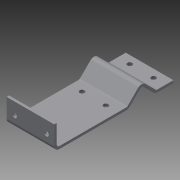
# Autodesk Inventor part: laserholder
Saved by Autodesk Inventor 2014 SP2 (Build 180246200, 246)
## iProperties
Created: 2016-05-15
Part Number: laserholder
Material: Generic
Document SubType Name: Sheet Metal
Designer: cruiser
Density: 1 g/cm^3
Sheet Metal Rule: Default_mm
Appearance: Default
Flat Pattern Width: 9.30164 cm
Flat Pattern Length: 3 cm
Flat Pattern Area: 27.9049 cm^2
Sheet Metal Width: 93.016 mm
Sheet Metal Length: 30.000 mm
Sheet Metal Area: 2790.493 mm^2
Author: cruiser
Autodesk Inventor part; units mm, degrees
ref_plane "YZ Plane" through (0, 0, 0) normal (1, 0, 0) x (0, 1, 0)
ref_plane "XZ Plane" through (0, 0, 0) normal (0, 1, 0) x (-1, 0, 0)
ref_plane "XY Plane" through (0, 0, 0) normal (0, 0, 1) x (1, 0, 0)
sketch "Sketch1" plane through (0, 0, 0) normal (0, 1, 0) x (-1, 0, 0)
  line L0 (15, -7.5) -> (-15, -7.5)
  line L1 (-15, -7.5) -> (-15, 7.5)
  line L2 (-15, 7.5) -> (15, 7.5)
  line L3 (15, 7.5) -> (15, -7.5)
  line L4 (15, -7.5) -> (-15, 7.5) construction
  line L5 (-15, -7.5) -> (15, 7.5) construction
  point P0 (0, 0)
  dimension "d10" = 30
  dimension "d11" = 15
  measures "d10" distance of L1.end L2.end
  measures "d11" distance of L0.end L1.end
extrude "Plate1" add sketch "Sketch1" along normal blind 1.5875
sketch "Sketch3" plane through (15, 0, 7.5) normal (1, 0, 0) x (0, 0, -1)
  line L0 (15, 0) -> (15, 1.5875)
  line L1 (15, 0) -> (15, 46.5147)
  line L2 (15, 0) -> (0, 0)
  line L3 (15, 63.4853) -> (15, 75)
  line L4 (6.5147, 55) -> (15, 46.5147)
  line L5 (15, 63.4853) -> (6.5147, 55)
  point P0 (7.5, 0)
  point P1 (15, 55)
  dimension "d48" = 75
  dimension "d91" = 55
  dimension "d92" = 0
  dimension "d94" = 90
  dimension "d95" = 135
  dimension "d96" = 6
  dimension "d97" = 6
  measures "d48" distance of L0.start L3.end
  measures "d91" distance from line of L2 point (15, 55)
  measures "d92" distance from line of L1 point (15, 55)
  measures "d94" angle of L5 L4
  measures "d95" angle of L3 L5
  measures "d96" distance from line of L4 point (15, 55)
  measures "d97" distance from line of L5 point (15, 55)
contour flange "Contour Flange4" sketch "Sketch3" thickness 1.5875 bend radius 1.5875 curves L1 L4 L5 L3 edges at (0, 1.5875, -7.5) running between points at (15, 1.5875, -7.5) (-15, 1.5875, -7.5)
bend "Bend4"
corner "Corner4"
sketch "Sketch4" plane through (-15, 75, -5.9125) normal (0, 0, 1) x (1, 0, 0)
  line L0 (0, -10.1996) -> (30, -10.1996) projected
  line L1 (30, 0) -> (0, 0) projected
  line L2 (0, 0) -> (0, -10.1996) projected
  circle A0 centre (7.5, -5) radius 1.5
  line L3 (15, 0) -> (15, -10.1996)
  circle A1 centre (22.5, -5) radius 1.5
  point P0 (15, -75)
  dimension "d50" = 3
  dimension "d52" = 5
  dimension "d53" = 7.5
  constraints: 2 centre point, 2 end point, 2 midpoint, 1 symmetric about line, 1 other
  measures "d50" diameter of A0
  measures "d52" distance from line of L1 A0.centre
  measures "d53" distance from line of L2 A0.centre
extrude "Cut1" cut sketch "Sketch4" against normal blind 1.5875 contours A0 | A1
sketch "Sketch9" plane through (-15, 45.1996, -5.9125) normal (0, 0, 1) x (1, 0, 0)
  line L0 (0, 0) -> (30, 0) projected
  line L1 (0, 0) -> (0, -42.0246) projected
  line L2 (0, -42.0246) -> (30, -42.0246) projected
  line L3 (30, 0) -> (30, -42.0246) projected
  circle A0 centre (7.5, -5.1996) radius 1.5
  line L4 (15, -42.0246) -> (15, 0)
  line L5 (0, -5.1996) -> (30, -5.1996)
  circle A1 centre (22.5, -5.1996) radius 1.5
  circle A2 centre (22.5, 24.8004) radius 1.5 projected
  point P0 (15, -45.1996)
  dimension "d79" = 3
  dimension "d81" = 7.5
  dimension "d84" = 30
  constraints: 4 end point, 3 point on line, 2 centre point, 2 midpoint, 1 perpendicular, 1 symmetric about line, 1 other
  measures "d79" diameter of A0
  measures "d81" distance from line of L1 A0.centre
  measures "d84" distance from line of A2.centre L5
extrude "Cut4" cut sketch "Sketch9" against normal blind 1.5875 contours L5 A0 | A0 L5 | A1 L5 | L5 A1
sketch "Sketch8" plane through (0, 0, 0) normal (0, -1, 0) x (1, 0, 0)
  line L0 (0, 0) -> (-15, 0)
  line L1 (-15, 0) -> (-15, 7.5)
  line L2 (-15, 7.5) -> (0, 7.5)
  line L3 (0, 7.5) -> (0, 0)
  circle A0 centre (-10, 0) radius 1.5
  circle A1 centre (10, 0) radius 1.5
  dimension "d75" = 3
  dimension "d76" = 5
  constraints: 8 end point, 2 centre point, 2 parallel, 1 horizontal, 1 perpendicular, 1 point on line, 1 symmetric about line, 1 other
  measures "d75" diameter of A0
  measures "d76" distance from line of L1 A0.centre
extrude "Cut3" cut sketch "Sketch8" against normal blind 1.5875 contours A0 L0 | L0 A0 | A1
equation "\"d10\" = laser_x"
equation "\"d11\" = laser_y"
equation "\"d48\" = laser_z"
equation "\"d50\" = m3_diameter"
equation "\"d53\" = 0.25 * laser_x"
equation "\"d54\" = Thickness"
equation "\"d79\" = m3_diameter"
equation "\"d81\" = 0.25 * laser_x"
equation "\"d82\" = Thickness"
equation "\"d75\" = m3_diameter"
equation "\"d76\" = 0.166667 * laser_x"
equation "\"d77\" = Thickness"
equation "\"Thickness\" = sm_thickness"
equation "\"d36\" = BendReliefWidth"
equation "\"d37\" = BendReliefDepth"
equation "\"d38\" = MinimumRemnant"
equation "\"d39\" = BendRadius"
equation "\"d40\" = BendRadius"
equation "\"d42\" = CornerReliefSize"
equation "\"d43\" = GapSize"
equation "\"d44\" = JacobiRadiusSize"
equation "\"BendRadius\" = Thickness"
equation "\"BendReliefWidth\" = Thickness"
equation "\"BendReliefDepth\" = 0.5 * Thickness"
equation "\"CornerReliefSize\" = 4 * Thickness"
equation "\"MinimumRemnant\" = 2 * Thickness"
equation "\"TransitionRadius\" = BendRadius"
equation "\"JacobiRadiusSize\" = BendRadius"
equation "\"GapSize\" = Thickness"
equation "\"d0\" = BendRadius"
equation "\"sm_thickness\" = 1.5875"
equation "\"very_thick_acrylic\" = 9.45"
equation "\"thick_acrylic\" = 5.88"
equation "\"thin_acrylic\" = 3.15"
equation "\"clear_acrylic\" = 3.15"
equation "\"wood_thickness\" = 6.72"
equation "\"m3_diameter\" = 3"
equation "\"m3_head\" = 6"
equation "\"m4_diameter\" = 4"
equation "\"m5_diameter\" = 5"
equation "\"m5_head\" = 10.3"
equation "\"brass_insert_drill\" = 4"
equation "\"m5_brass_insert_drill\" = 6.7"
equation "\"m3_press_nut_drill\" = 4.5"
equation "\"m5_press_nut_drill\" = 6.5"
equation "\"stepper_screw_space\" = 35"
equation "\"stepper_shaft_diameter\" = 5"
equation "\"stepper_body_diameter\" = 28"
equation "\"laser_body_diameter\" = 12"
equation "\"carrier_y\" = 251"
equation "\"carrier_z\" = 12"
equation "\"visor_x\" = 253.925"
equation "\"visor_y\" = 85.6"
equation "\"window_z\" = 332.225"
equation "\"window_y\" = 93.75"
equation "\"window_overlap\" = 48"
equation "\"acrylic_into_frame\" = 5"
equation "\"door_x\" = 251"
equation "\"door_z\" = 332.225"
equation "\"door_overlap\" = 48"
equation "\"reservoir_x\" = 201"
equation "\"reservoir_y\" = 201"
equation "\"linear_bearing_spacing\" = 271"
equation "\"tray_border\" = 25"
equation "\"tray_x\" = 251"
equation "\"tray_y\" = 251"
equation "\"bed_z\" = 25"
equation "\"crane_z2\" = 12"
equation "\"end_stop_spacing\" = 19"
equation "\"thumb_nut_offset_y\" = 0"
equation "\"thumb_nut_diameter\" = 7"
equation "\"z_min_from_center\" = 115"
equation "\"frame_top_z\" = 385"
equation "\"frame_bottom_z\" = 275"
equation "\"frame_total_z\" = 661.5875"
equation "\"frame_border\" = 48.0375"
equation "\"frame_foot_z\" = 12"
equation "\"frame_tilt\" = 1deg"
equation "\"subframe_x\" = 66"
equation "\"subframe_y_offset\" = 27.5"
equation "\"laser_y_offset\" = 19.4"
equation "\"laser_diameter\" = 12"
equation "\"laser_z_offset\" = 55"
equation "\"laser_y\" = 15"
equation "\"laser_z\" = 75"
equation "\"laser_x\" = 30"
equation "\"t_galvo_frame\" = 6.72"
equation "\"galvo_frame_x\" = 66"
equation "\"galvo_frame_z\" = 85"
equation "\"galvo_frame_y_offset\" = 27.5"
equation "\"drawer_x\" = 257.3"
equation "\"drawer_y\" = 90.3375"
equation "\"drawer_z\" = 278.175"
equation "\"drawer_support_from_top\" = 48"
equation "\"nema17_x\" = 43"
equation "\"laser_gap\" = 1"
equation "\"frame_screw_from_center\" = 25"
equation "\"drawer_screw_from_center\" = 55"
equation "\"frame_face_y\" = 45"
equation "\"switch_spacing\" = 19"
equation "\"subframe_y\" = 55"
equation "\"al_thickness\" = 1.5875"
equation "\"rivet_diameter\" = 3.3"
equation "\"bend_factor\" = 2.26205"
equation "\"al_bend\" = 3.591"
equation "\"sm_bend\" = 3.591"
equation "\"frame_x\" = 353.375"
equation "\"carrier_z2\" = 25"
equation "\"carrier_y2\" = 76.825"
body "Solid1"
